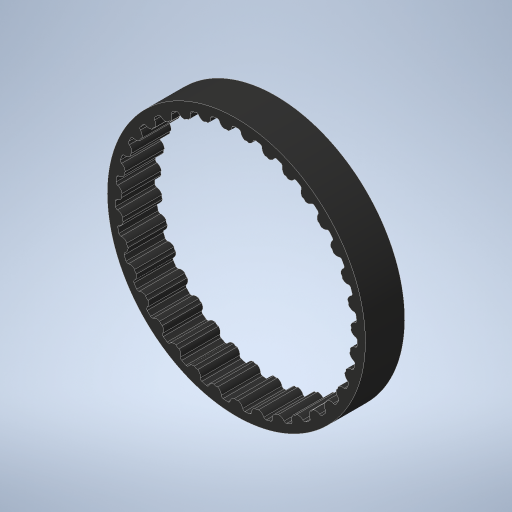
# Autodesk Inventor part: belt tooth
Saved by Autodesk Inventor 2023.3 (Build 273359000, 359)
## iProperties
Created: 2024-02-03
Part Number: belt tooth
Material: Rubber, Silicone
Document SubType Name: Modeling
Designer: mavericks
Density: 1.25 g/cm^3
Appearance: Rubber - Black
Author: mavericks
Autodesk Inventor part; units mm, degrees
ref_plane "YZ Plane" through (0, 0, 0) normal (1, 0, 0) x (0, 1, 0)
ref_plane "XZ Plane" through (0, 0, 0) normal (0, 1, 0) x (-1, 0, 0)
ref_plane "XY Plane" through (0, 0, 0) normal (0, 0, 1) x (1, 0, 0)
sketch "Sketch1" plane through (0, 0, 0) normal (0, 0, 1) x (1, 0, 0)
  line L0 (3.873, 1.9) -> (5, 1.9) construction
  arc A0 (3.3889, 2.275) -> (3.873, 1.9) centre (3.873, 2.4) ccw
  arc A1 (3.3889, 2.275) -> (2.3532, 3.341) centre (1.9365, 1.9) ccw
  arc A2 (1.5198, 3.341) -> (2.3532, 3.341) centre (1.9365, 4.0627) ccw
  arc A3 (1.5198, 3.341) -> (0.4841, 2.275) centre (1.9365, 1.9) ccw
  arc A4 (0, 1.9) -> (0.4841, 2.275) centre (0, 2.4) ccw
  line L1 (0, 0) -> (6.35, 0) construction
  line L2 (0, 1.9) -> (0, 0)
  line L3 (3.873, 1.9) -> (3.873, 0)
  line L4 (3.873, 0) -> (0, 0)
  dimension "d1" = 1.127
  dimension "d2" = 0.5
  dimension "d3" = 1.5
  dimension "d4" = 0.8333
  dimension "d5" = 1.5
  dimension "d6" = 0.5
  dimension "d7" = 1.9
  dimension "d8" = 2.4
  dimension "d9" = 1.9365
  dimension "d10" = 1.9365
  dimension "d11" = 1.6626
  dimension "d12" = 0.5
  dimension "d13" = 1.9
  dimension "d14" = 0
  dimension "d15" = 6.35
  dimension "d16" = 0.4841
  dimension "d17" = 1.0357
  dimension "d18" = 0.375
  dimension "d19" = 1.066
  dimension "Height_of_Tooth" = 3.341
  constraints: 10 end point, 10 point on circle, 5 centre point, 2 perpendicular, 1 coincident, 1 horizontal, 1 point on line
  measures "d1" distance of L0.start L0.end
  measures "d2" radius of A0
  measures "d3" radius of A1
  measures "d4" radius of A2
  measures "d5" radius of A3
  measures "d6" radius of A4
  measures "d7" distance between parallel lines of L1 L0
  measures "d8" distance from line of L1 A4.centre
  measures "d9" horizontal distance of A2.centre A4.centre
  measures "d10" horizontal distance of A0.centre A2.centre
  measures "d11" vertical distance of A2.centre A0.centre
  measures "d12" vertical distance of A1.centre A0.centre
  measures "d13" distance from line of L1 A1.centre
  measures "d14" horizontal distance of L1.start A4.centre
  measures "d15" distance of L1.start L1.end
  measures "d16" horizontal distance of L0.start A0.start
  measures "d17" horizontal distance of A3.end A3.start
  measures "d18" vertical distance of L2.start A3.end
  measures "d19" vertical distance of A3.end A3.start
  measures "Height_of_Tooth" distance from line of L1 A3.start
extrude "Extrusion1" add sketch "Sketch1" along normal mid plane 9
ref_plane "Work Plane1" through (0, 29.5226, 4.5) normal (0, -1, 0) x (1, 0, 0)
sketch "Sketch2" plane through (0, 29.5226, 4.5) normal (0, -1, 0) x (1, 0, 0)
  line L0 (1.5198, -9) -> (1.5198, 0) construction
  line L1 (2.3532, 0) -> (2.3532, 0) construction
  line L2 (2.3532, 0) -> (2.3532, -9) construction
  line L3 (1.5198, -9) -> (2.3532, -9) construction
  line L4 (3.873, -9) -> (0, -9) construction
  line L5 (1.9365, -9) -> (1.9365, 0)
  line L6 (2.3532, 0) -> (2.3532, 0) construction
  point P0 (0, -4.5)
  constraints: 2 end point, 1 midpoint, 1 point on line
pattern_circular "Circular Pattern1" count 35 over 360 about axis through (1.9365, 29.5226, -4.5) along (0, 0, 1) of "Extrusion1"
sketch "Sketch3" plane through (0, 0, 4.5) normal (0, 0, 1) x (1, 0, 0)
  arc A0 (3.3889, 2.275) -> (2.3532, 3.341) centre (1.9365, 1.9) ccw construction
  arc A1 (3.3889, 2.275) -> (3.873, 1.9) centre (3.873, 2.4) ccw construction
  line L0 (3.873, 1.9) -> (3.873, 0) construction
  line L1 (3.873, 0) -> (0, 0) construction
  line L2 (0, 0) -> (0, 1.9) construction
  arc A2 (0, 1.9) -> (0.4841, 2.275) centre (0, 2.4) ccw construction
  arc A3 (1.5198, 3.341) -> (0.4841, 2.275) centre (1.9365, 1.9) ccw construction
  arc A4 (1.5198, 3.341) -> (2.3532, 3.341) centre (1.9365, 4.0627) ccw construction
  arc A5 (8.2308, 2.9722) -> (7.0214, 3.8361) centre (6.8687, 2.3439) ccw construction
  arc A6 (8.2308, 2.9722) -> (8.7741, 2.6897) centre (8.6848, 3.1816) ccw construction
  line L3 (8.7741, 2.6897) -> (9.1133, 0.8202) construction
  line L4 (9.1133, 0.8202) -> (5.3026, 0.1287) construction
  line L5 (5.3026, 0.1287) -> (4.9633, 1.9981) construction
  arc A7 (4.9633, 1.9981) -> (5.3727, 2.4535) centre (4.874, 2.4901) ccw construction
  arc A8 (6.2014, 3.6873) -> (5.3727, 2.4535) centre (6.8687, 2.3439) ccw construction
  arc A9 (6.2014, 3.6873) -> (7.0214, 3.8361) centre (6.4825, 4.4718) ccw construction
  arc A10 (12.8704, 4.5228) -> (11.5262, 5.1568) centre (11.6424, 3.6614) ccw construction
  arc A11 (12.8704, 4.5228) -> (13.4554, 4.3418) centre (13.2797, 4.8099) ccw construction
  line L6 (13.4554, 4.3418) -> (14.123, 2.5629) construction
  line L7 (14.123, 2.5629) -> (10.497, 1.2021) construction
  line L8 (10.497, 1.2021) -> (9.8294, 2.9809) construction
  arc A12 (9.8294, 2.9809) -> (10.1509, 3.5021) centre (9.6537, 3.449) ccw construction
  arc A13 (10.746, 4.864) -> (10.1509, 3.5021) centre (11.6424, 3.6614) ccw construction
  arc A14 (10.746, 4.864) -> (11.5262, 5.1568) centre (10.8825, 5.6861) ccw construction
  arc A15 (17.1585, 6.8768) -> (15.7227, 7.2607) centre (16.1041, 5.81) ccw construction
  arc A16 (17.1585, 6.8768) -> (17.7665, 6.8032) centre (17.51, 7.2325) ccw construction
  line L9 (17.7665, 6.8032) -> (18.741, 5.1722) construction
  line L10 (18.741, 5.1722) -> (15.4162, 3.1857) construction
  line L11 (15.4162, 3.1857) -> (14.4417, 4.8168) construction
  arc A17 (14.4417, 4.8168) -> (14.665, 5.387) centre (14.1853, 5.246) ccw construction
  arc A18 (15.0073, 6.8333) -> (14.665, 5.387) centre (16.1041, 5.81) ccw construction
  arc A19 (15.0073, 6.8333) -> (15.7227, 7.2607) centre (14.9949, 7.6665) ccw construction
  arc A20 (20.9575, 9.9588) -> (19.4762, 10.0801) centre (20.1105, 8.7208) ccw construction
  arc A21 (20.9575, 9.9588) -> (21.5688, 9.9949) centre (21.2398, 10.3714) ccw construction
  line L12 (21.5688, 9.9949) -> (22.8189, 8.5641) construction
  line L13 (22.8189, 8.5641) -> (19.9022, 6.0159) construction
  line L14 (19.9022, 6.0159) -> (18.6522, 7.4467) construction
  arc A22 (18.6522, 7.4467) -> (18.77, 8.0476) centre (18.3232, 7.8233) ccw construction
  arc A23 (18.8486, 9.5318) -> (18.77, 8.0476) centre (20.1105, 8.7208) ccw construction
  arc A24 (18.8486, 9.5318) -> (19.4762, 10.0801) centre (18.6876, 10.3494) ccw construction
  arc A25 (24.1451, 13.6695) -> (22.6659, 13.5244) centre (23.5327, 12.3002) ccw construction
  arc A26 (24.1451, 13.6695) -> (24.7401, 13.8142) centre (24.3492, 14.1259) ccw construction
  line L15 (24.7401, 13.8142) -> (26.2256, 12.6296) construction
  line L16 (26.2256, 12.6296) -> (23.8108, 9.6016) construction
  line L17 (23.8108, 9.6016) -> (22.3253, 10.7862) construction
  arc A27 (22.3253, 10.7862) -> (22.334, 11.3985) centre (21.9344, 11.0979) ccw construction
  arc A28 (22.1463, 12.8729) -> (22.334, 11.3985) centre (23.5327, 12.3002) ccw construction
  arc A29 (22.1463, 12.8729) -> (22.6659, 13.5244) centre (21.8419, 13.6486) ccw construction
  arc A30 (26.6188, 17.8898) -> (25.1894, 17.4829) centre (26.2608, 16.4331) ccw construction
  arc A31 (26.6188, 17.8898) -> (27.1785, 18.1384) centre (26.7382, 18.3753) ccw construction
  line L18 (27.1785, 18.1384) -> (28.8516, 17.238) construction
  line L19 (28.8516, 17.238) -> (27.0163, 13.8275) construction
  line L20 (27.0163, 13.8275) -> (25.3432, 14.7278) construction
  arc A32 (25.3432, 14.7278) -> (25.2424, 15.3319) centre (24.9029, 14.9648) ccw construction
  arc A33 (24.7945, 16.749) -> (25.2424, 15.3319) centre (26.2608, 16.4331) ccw construction
  arc A34 (24.7945, 16.749) -> (25.1894, 17.4829) centre (24.3564, 17.4579) ccw construction
  arc A35 (28.2993, 22.4839) -> (26.9655, 21.8283) centre (28.2071, 20.9867) ccw construction
  arc A36 (28.2993, 22.4839) -> (28.8056, 22.8285) centre (28.33, 22.983) ccw construction
  line L21 (28.8056, 22.8285) -> (30.6126, 22.2413) construction
  line L22 (30.6126, 22.2413) -> (29.4157, 18.5579) construction
  line L23 (29.4157, 18.5579) -> (27.6087, 19.145) construction
  arc A37 (27.6087, 19.145) -> (27.4017, 19.7213) centre (27.1332, 19.2995) ccw construction
  arc A38 (26.7079, 21.0358) -> (27.4017, 19.7213) centre (28.2071, 20.9867) ccw construction
  arc A39 (26.7079, 21.0358) -> (26.9655, 21.8283) centre (26.1503, 21.655) ccw construction
  arc A40 (29.1324, 27.3043) -> (27.9371, 26.421) centre (29.3091, 25.8147) ccw construction
  arc A41 (29.1324, 27.3043) -> (29.569, 27.7337) centre (29.0736, 27.8008) ccw construction
  line L24 (29.569, 27.7337) -> (31.4518, 27.4786) construction
  line L25 (31.4518, 27.4786) -> (30.932, 23.6407) construction
  line L26 (30.932, 23.6407) -> (29.0492, 23.8958) construction
  arc A42 (29.0492, 23.8958) -> (28.7425, 24.4258) centre (28.5537, 23.9629) ccw construction
  arc A43 (27.8252, 25.5953) -> (28.7425, 24.4258) centre (29.3091, 25.8147) ccw construction
  arc A44 (27.8252, 25.5953) -> (27.9371, 26.421) centre (27.166, 26.105) ccw construction
  arc A45 (29.0915, 32.196) -> (28.0731, 31.1135) centre (29.5313, 30.7619) ccw construction
  arc A46 (29.0915, 32.196) -> (29.4444, 32.6964) centre (28.9449, 32.674) ccw construction
  line L27 (29.4444, 32.6964) -> (31.3425, 32.7817) construction
  line L28 (31.3425, 32.7817) -> (31.5162, 28.9126) construction
  line L29 (31.5162, 28.9126) -> (29.6182, 28.8273) construction
  arc A47 (29.6182, 28.8273) -> (29.2218, 29.2942) centre (29.1187, 28.8049) ccw construction
  arc A48 (28.1105, 30.281) -> (29.2218, 29.2942) centre (29.5313, 30.7619) ccw construction
  arc A49 (28.1105, 30.281) -> (28.0731, 31.1135) centre (27.3708, 30.6649) ccw construction
  arc A50 (28.1778, 37.0017) -> (27.369, 35.7548) centre (28.8665, 35.6692) ccw construction
  arc A51 (28.1778, 37.0017) -> (28.4356, 37.5571) centre (27.9482, 37.4459) ccw construction
  line L30 (28.4356, 37.5571) -> (30.288, 37.9799) construction
  line L31 (30.288, 37.9799) -> (31.1498, 34.2041) construction
  line L32 (31.1498, 34.2041) -> (29.2974, 33.7813) construction
  arc A52 (29.2974, 33.7813) -> (28.8241, 34.1698) centre (28.81, 33.67) ccw construction
  arc A53 (27.5544, 34.9423) -> (28.8241, 34.1698) centre (28.8665, 35.6692) ccw construction
  arc A54 (27.5544, 34.9423) -> (27.369, 35.7548) centre (26.7581, 35.188) ccw construction
  arc A55 (26.4206, 41.5671) -> (25.8475, 40.1958) centre (27.3362, 40.379) ccw construction
  arc A56 (26.4206, 41.5671) -> (26.5751, 42.1596) centre (26.1154, 41.9631) ccw construction
  line L33 (26.5751, 42.1596) -> (28.3223, 42.9064) construction
  line L34 (28.3223, 42.9064) -> (29.8444, 39.3451) construction
  line L35 (29.8444, 39.3451) -> (28.0973, 38.5983) construction
  arc A57 (28.0973, 38.5983) -> (27.5622, 38.8961) centre (27.6376, 38.4018) ccw construction
  arc A58 (26.175, 39.4295) -> (27.5622, 38.8961) centre (27.3362, 40.379) ccw construction
  arc A59 (26.175, 39.4295) -> (25.8475, 40.1958) centre (25.3476, 39.529) ccw construction
  arc A60 (23.8765, 45.7453) -> (23.5574, 44.2937) centre (24.9896, 44.7398) ccw construction
  arc A61 (23.8765, 45.7453) -> (23.9228, 46.3559) centre (23.5055, 46.0805) ccw construction
  line L36 (23.9228, 46.3559) -> (25.5085, 47.4027) construction
  line L37 (25.5085, 47.4027) -> (27.6421, 44.1704) construction
  line L38 (27.6421, 44.1704) -> (26.0564, 43.1237) construction
  arc A62 (26.0564, 43.1237) -> (25.4767, 43.3211) centre (25.6391, 42.8482) ccw construction
  arc A63 (24.0165, 43.5982) -> (25.4767, 43.3211) centre (24.9896, 44.7398) ccw construction
  arc A64 (24.0165, 43.5982) -> (23.5574, 44.2937) centre (23.1847, 43.5484) ccw construction
  arc A65 (20.6272, 49.4022) -> (20.5725, 47.9169) centre (21.902, 48.6115) ccw construction
  arc A66 (20.6272, 49.4022) -> (20.5637, 50.0112) centre (20.2023, 49.6657) ccw construction
  line L39 (20.5637, 50.0112) -> (21.937, 51.3242) construction
  line L40 (21.937, 51.3242) -> (24.6135, 48.5249) construction
  line L41 (24.6135, 48.5249) -> (23.2402, 47.2119) construction
  arc A67 (23.2402, 47.2119) -> (22.6346, 47.3026) centre (22.8788, 46.8663) ccw construction
  arc A68 (21.1484, 47.3146) -> (22.6346, 47.3026) centre (21.902, 48.6115) ccw construction
  arc A69 (21.1484, 47.3146) -> (20.5725, 47.9169) centre (20.3388, 47.117) ccw construction
  arc A70 (16.7772, 52.4201) -> (16.9886, 50.9489) centre (18.1726, 51.8698) ccw construction
  arc A71 (16.7772, 52.4201) -> (16.606, 53.008) centre (16.3121, 52.6035) ccw construction
  line L42 (16.606, 53.008) -> (17.7228, 54.5451) construction
  line L43 (17.7228, 54.5451) -> (20.8561, 52.2686) construction
  line L44 (20.8561, 52.2686) -> (19.7393, 50.7315) construction
  arc A72 (19.7393, 50.7315) -> (19.1272, 50.7127) centre (19.4454, 50.327) ccw construction
  arc A73 (17.6628, 50.4591) -> (19.1272, 50.7127) centre (18.1726, 51.8698) ccw construction
  arc A74 (17.6628, 50.4591) -> (16.9886, 50.9489) centre (16.9015, 50.1201) ccw construction
  arc A75 (12.4502, 54.702) -> (12.9209, 53.2922) centre (13.9215, 54.4097) ccw construction
  arc A76 (12.4502, 54.702) -> (12.1768, 55.2499) centre (11.9598, 54.7994) ccw construction
  line L45 (12.1768, 55.2499) -> (13.0011, 56.9618) construction
  line L46 (13.0011, 56.9618) -> (16.4906, 55.2813) construction
  line L47 (16.4906, 55.2813) -> (15.6662, 53.5695) construction
  arc A77 (15.6662, 53.5695) -> (15.0673, 53.4417) centre (15.4493, 53.119) ccw construction
  arc A78 (13.6717, 52.9307) -> (15.0673, 53.4417) centre (13.9215, 54.4097) ccw construction
  arc A79 (13.6717, 52.9307) -> (12.9209, 53.2922) centre (12.9831, 52.4612) ccw construction
  arc A80 (7.7853, 56.1747) -> (8.5001, 54.8716) centre (9.2851, 56.1498) ccw construction
  arc A81 (7.7853, 56.1747) -> (7.4184, 56.6649) centre (7.2854, 56.183) ccw construction
  line L48 (7.4184, 56.6649) -> (7.9239, 58.4965) construction
  line L49 (7.9239, 58.4965) -> (11.6573, 57.4661) construction
  line L50 (11.6573, 57.4661) -> (11.1518, 55.6346) construction
  arc A82 (11.1518, 55.6346) -> (10.5854, 55.4019) centre (11.0188, 55.1526) ccw construction
  arc A83 (9.3034, 54.6499) -> (10.5854, 55.4019) centre (9.2851, 56.1498) ccw construction
  arc A84 (9.3034, 54.6499) -> (8.5001, 54.8716) centre (8.7098, 54.065) ccw construction
  arc A85 (2.9324, 56.7907) -> (3.8684, 55.6362) centre (4.4126, 57.034) ccw construction
  arc A86 (2.9324, 56.7907) -> (2.4839, 57.2076) centre (2.439, 56.7096) ccw construction
  line L51 (2.4839, 57.2076) -> (2.6542, 59.0999) construction
  line L52 (2.6542, 59.0999) -> (6.5116, 58.7528) construction
  line L53 (6.5116, 58.7528) -> (6.3413, 56.8604) construction
  arc A87 (6.3413, 56.8604) -> (5.8255, 56.5303) centre (6.2964, 56.3624) ccw construction
  arc A88 (4.6984, 55.5615) -> (5.8255, 56.5303) centre (4.4126, 57.034) ccw construction
  arc A89 (4.6984, 55.5615) -> (3.8684, 55.6362) centre (4.2187, 54.8801) ccw construction
  arc A90 (-1.9525, 56.5303) -> (-0.8254, 55.5615) centre (-0.5396, 57.034) ccw construction
  arc A91 (-1.9525, 56.5303) -> (-2.4683, 56.8604) centre (-2.4235, 56.3624) ccw construction
  line L54 (-2.4683, 56.8604) -> (-2.6386, 58.7528) construction
  line L55 (-2.6386, 58.7528) -> (1.2188, 59.0999) construction
  line L56 (1.2188, 59.0999) -> (1.3891, 57.2076) construction
  arc A92 (1.3891, 57.2076) -> (0.9406, 56.7907) centre (1.4339, 56.7096) ccw construction
  arc A93 (0.0046, 55.6362) -> (0.9406, 56.7907) centre (-0.5396, 57.034) ccw construction
  arc A94 (0.0046, 55.6362) -> (-0.8254, 55.5615) centre (-0.3457, 54.8801) ccw construction
  arc A95 (-6.7124, 55.4019) -> (-5.4304, 54.6499) centre (-5.4121, 56.1498) ccw construction
  arc A96 (-6.7124, 55.4019) -> (-7.2788, 55.6346) centre (-7.1458, 55.1526) ccw construction
  line L57 (-7.2788, 55.6346) -> (-7.7843, 57.4661) construction
  line L58 (-7.7843, 57.4661) -> (-4.0509, 58.4965) construction
  line L59 (-4.0509, 58.4965) -> (-3.5454, 56.6649) construction
  arc A97 (-3.5454, 56.6649) -> (-3.9123, 56.1747) centre (-3.4124, 56.183) ccw construction
  arc A98 (-4.6271, 54.8716) -> (-3.9123, 56.1747) centre (-5.4121, 56.1498) ccw construction
  arc A99 (-4.6271, 54.8716) -> (-5.4304, 54.6499) centre (-4.8368, 54.065) ccw construction
  arc A100 (-11.1943, 53.4417) -> (-9.7987, 52.9307) centre (-10.0485, 54.4097) ccw construction
  arc A101 (-11.1943, 53.4417) -> (-11.7932, 53.5695) centre (-11.5763, 53.119) ccw construction
  line L60 (-11.7932, 53.5695) -> (-12.6176, 55.2813) construction
  line L61 (-12.6176, 55.2813) -> (-9.1282, 56.9618) construction
  line L62 (-9.1282, 56.9618) -> (-8.3038, 55.2499) construction
  arc A102 (-8.3038, 55.2499) -> (-8.5773, 54.702) centre (-8.0868, 54.7994) ccw construction
  arc A103 (-9.0479, 53.2922) -> (-8.5773, 54.702) centre (-10.0485, 54.4097) ccw construction
  arc A104 (-9.0479, 53.2922) -> (-9.7987, 52.9307) centre (-9.1102, 52.4612) ccw construction
  arc A105 (-15.2542, 50.7127) -> (-13.7898, 50.4591) centre (-14.2997, 51.8698) ccw construction
  arc A106 (-15.2542, 50.7127) -> (-15.8663, 50.7315) centre (-15.5724, 50.327) ccw construction
  line L63 (-15.8663, 50.7315) -> (-16.9831, 52.2686) construction
  line L64 (-16.9831, 52.2686) -> (-13.8498, 54.5451) construction
  line L65 (-13.8498, 54.5451) -> (-12.733, 53.008) construction
  arc A107 (-12.733, 53.008) -> (-12.9043, 52.4201) centre (-12.4391, 52.6035) ccw construction
  arc A108 (-13.1156, 50.9489) -> (-12.9043, 52.4201) centre (-14.2997, 51.8698) ccw construction
  arc A109 (-13.1156, 50.9489) -> (-13.7898, 50.4591) centre (-13.0285, 50.1201) ccw construction
  arc A110 (-18.7616, 47.3026) -> (-17.2754, 47.3146) centre (-18.029, 48.6115) ccw construction
  arc A111 (-18.7616, 47.3026) -> (-19.3672, 47.2119) centre (-19.0058, 46.8663) ccw construction
  line L66 (-19.3672, 47.2119) -> (-20.7405, 48.5249) construction
  line L67 (-20.7405, 48.5249) -> (-18.0641, 51.3242) construction
  line L68 (-18.0641, 51.3242) -> (-16.6907, 50.0112) construction
  arc A112 (-16.6907, 50.0112) -> (-16.7543, 49.4022) centre (-16.3293, 49.6657) ccw construction
  arc A113 (-16.6995, 47.9169) -> (-16.7543, 49.4022) centre (-18.029, 48.6115) ccw construction
  arc A114 (-16.6995, 47.9169) -> (-17.2754, 47.3146) centre (-16.4658, 47.117) ccw construction
  arc A115 (-21.6037, 43.3211) -> (-20.1435, 43.5982) centre (-21.1166, 44.7398) ccw construction
  arc A116 (-21.6037, 43.3211) -> (-22.1834, 43.1237) centre (-21.7661, 42.8482) ccw construction
  line L69 (-22.1834, 43.1237) -> (-23.7691, 44.1704) construction
  line L70 (-23.7691, 44.1704) -> (-21.6355, 47.4027) construction
  line L71 (-21.6355, 47.4027) -> (-20.0498, 46.3559) construction
  arc A117 (-20.0498, 46.3559) -> (-20.0035, 45.7453) centre (-19.6325, 46.0805) ccw construction
  arc A118 (-19.6845, 44.2937) -> (-20.0035, 45.7453) centre (-21.1166, 44.7398) ccw construction
  arc A119 (-19.6845, 44.2937) -> (-20.1435, 43.5982) centre (-19.3117, 43.5484) ccw construction
  arc A120 (-23.6893, 38.8961) -> (-22.302, 39.4295) centre (-23.4633, 40.379) ccw construction
  arc A121 (-23.6893, 38.8961) -> (-24.2243, 38.5983) centre (-23.7646, 38.4018) ccw construction
  line L72 (-24.2243, 38.5983) -> (-25.9714, 39.3451) construction
  line L73 (-25.9714, 39.3451) -> (-24.4493, 42.9064) construction
  line L74 (-24.4493, 42.9064) -> (-22.7022, 42.1596) construction
  arc A122 (-22.7022, 42.1596) -> (-22.5476, 41.5671) centre (-22.2424, 41.9631) ccw construction
  arc A123 (-21.9745, 40.1958) -> (-22.5476, 41.5671) centre (-23.4633, 40.379) ccw construction
  arc A124 (-21.9745, 40.1958) -> (-22.302, 39.4295) centre (-21.4746, 39.529) ccw construction
  arc A125 (-24.9511, 34.1698) -> (-23.6814, 34.9423) centre (-24.9936, 35.6692) ccw construction
  arc A126 (-24.9511, 34.1698) -> (-25.4245, 33.7813) centre (-24.937, 33.67) ccw construction
  line L75 (-25.4245, 33.7813) -> (-27.2768, 34.2041) construction
  line L76 (-27.2768, 34.2041) -> (-26.415, 37.9799) construction
  line L77 (-26.415, 37.9799) -> (-24.5626, 37.5571) construction
  arc A127 (-24.5626, 37.5571) -> (-24.3048, 37.0017) centre (-24.0752, 37.4459) ccw construction
  arc A128 (-23.496, 35.7548) -> (-24.3048, 37.0017) centre (-24.9936, 35.6692) ccw construction
  arc A129 (-23.496, 35.7548) -> (-23.6814, 34.9423) centre (-22.8851, 35.188) ccw construction
  arc A130 (-25.3488, 29.2942) -> (-24.2375, 30.281) centre (-25.6583, 30.7619) ccw construction
  arc A131 (-25.3488, 29.2942) -> (-25.7452, 28.8273) centre (-25.2457, 28.8049) ccw construction
  line L78 (-25.7452, 28.8273) -> (-27.6433, 28.9126) construction
  line L79 (-27.6433, 28.9126) -> (-27.4695, 32.7817) construction
  line L80 (-27.4695, 32.7817) -> (-25.5714, 32.6964) construction
  arc A132 (-25.5714, 32.6964) -> (-25.2185, 32.196) centre (-25.0719, 32.674) ccw construction
  arc A133 (-24.2001, 31.1135) -> (-25.2185, 32.196) centre (-25.6583, 30.7619) ccw construction
  arc A134 (-24.2001, 31.1135) -> (-24.2375, 30.281) centre (-23.4978, 30.6649) ccw construction
  arc A135 (-24.8696, 24.4258) -> (-23.9523, 25.5953) centre (-25.4361, 25.8147) ccw construction
  arc A136 (-24.8696, 24.4258) -> (-25.1762, 23.8958) centre (-24.6807, 23.9629) ccw construction
  line L81 (-25.1762, 23.8958) -> (-27.059, 23.6407) construction
  line L82 (-27.059, 23.6407) -> (-27.5789, 27.4786) construction
  line L83 (-27.5789, 27.4786) -> (-25.6961, 27.7337) construction
  arc A137 (-25.6961, 27.7337) -> (-25.2595, 27.3043) centre (-25.2006, 27.8008) ccw construction
  arc A138 (-24.0641, 26.421) -> (-25.2595, 27.3043) centre (-25.4361, 25.8147) ccw construction
  arc A139 (-24.0641, 26.421) -> (-23.9523, 25.5953) centre (-23.293, 26.105) ccw construction
  arc A140 (-23.5287, 19.7213) -> (-22.835, 21.0358) centre (-24.3342, 20.9867) ccw construction
  arc A141 (-23.5287, 19.7213) -> (-23.7358, 19.145) centre (-23.2602, 19.2995) ccw construction
  line L84 (-23.7358, 19.145) -> (-25.5428, 18.5579) construction
  line L85 (-25.5428, 18.5579) -> (-26.7396, 22.2413) construction
  line L86 (-26.7396, 22.2413) -> (-24.9326, 22.8285) construction
  arc A142 (-24.9326, 22.8285) -> (-24.4263, 22.4839) centre (-24.457, 22.983) ccw construction
  arc A143 (-23.0925, 21.8283) -> (-24.4263, 22.4839) centre (-24.3342, 20.9867) ccw construction
  arc A144 (-23.0925, 21.8283) -> (-22.835, 21.0358) centre (-22.2774, 21.655) ccw construction
  arc A145 (-21.3694, 15.3319) -> (-20.9215, 16.749) centre (-22.3878, 16.4331) ccw construction
  arc A146 (-21.3694, 15.3319) -> (-21.4702, 14.7278) centre (-21.0299, 14.9648) ccw construction
  line L87 (-21.4702, 14.7278) -> (-23.1433, 13.8275) construction
  line L88 (-23.1433, 13.8275) -> (-24.9786, 17.238) construction
  line L89 (-24.9786, 17.238) -> (-23.3055, 18.1384) construction
  arc A147 (-23.3055, 18.1384) -> (-22.7459, 17.8898) centre (-22.8652, 18.3753) ccw construction
  arc A148 (-21.3164, 17.4829) -> (-22.7459, 17.8898) centre (-22.3878, 16.4331) ccw construction
  arc A149 (-21.3164, 17.4829) -> (-20.9215, 16.749) centre (-20.4834, 17.4579) ccw construction
  arc A150 (-18.461, 11.3985) -> (-18.2733, 12.8729) centre (-19.6597, 12.3002) ccw construction
  arc A151 (-18.461, 11.3985) -> (-18.4523, 10.7862) centre (-18.0614, 11.0979) ccw construction
  line L90 (-18.4523, 10.7862) -> (-19.9378, 9.6016) construction
  line L91 (-19.9378, 9.6016) -> (-22.3526, 12.6296) construction
  line L92 (-22.3526, 12.6296) -> (-20.8671, 13.8142) construction
  arc A152 (-20.8671, 13.8142) -> (-20.2721, 13.6695) centre (-20.4762, 14.1259) ccw construction
  arc A153 (-18.7929, 13.5244) -> (-20.2721, 13.6695) centre (-19.6597, 12.3002) ccw construction
  arc A154 (-18.7929, 13.5244) -> (-18.2733, 12.8729) centre (-17.9689, 13.6486) ccw construction
  arc A155 (-14.897, 8.0476) -> (-14.9756, 9.5318) centre (-16.2375, 8.7208) ccw construction
  arc A156 (-14.897, 8.0476) -> (-14.7792, 7.4467) centre (-14.4502, 7.8233) ccw construction
  line L93 (-14.7792, 7.4467) -> (-16.0293, 6.0159) construction
  line L94 (-16.0293, 6.0159) -> (-18.9459, 8.5641) construction
  line L95 (-18.9459, 8.5641) -> (-17.6958, 9.9949) construction
  arc A157 (-17.6958, 9.9949) -> (-17.0845, 9.9588) centre (-17.3668, 10.3714) ccw construction
  arc A158 (-15.6032, 10.0801) -> (-17.0845, 9.9588) centre (-16.2375, 8.7208) ccw construction
  arc A159 (-15.6032, 10.0801) -> (-14.9756, 9.5318) centre (-14.8146, 10.3494) ccw construction
  arc A160 (-10.792, 5.387) -> (-11.1344, 6.8333) centre (-12.2311, 5.81) ccw construction
  arc A161 (-10.792, 5.387) -> (-10.5687, 4.8168) centre (-10.3123, 5.246) ccw construction
  line L96 (-10.5687, 4.8168) -> (-11.5433, 3.1857) construction
  line L97 (-11.5433, 3.1857) -> (-14.868, 5.1722) construction
  line L98 (-14.868, 5.1722) -> (-13.8935, 6.8032) construction
  arc A162 (-13.8935, 6.8032) -> (-13.2856, 6.8768) centre (-13.637, 7.2325) ccw construction
  arc A163 (-11.8497, 7.2607) -> (-13.2856, 6.8768) centre (-12.2311, 5.81) ccw construction
  arc A164 (-11.8497, 7.2607) -> (-11.1344, 6.8333) centre (-11.1219, 7.6665) ccw construction
  arc A165 (-6.2779, 3.5021) -> (-6.873, 4.864) centre (-7.7694, 3.6614) ccw construction
  arc A166 (-6.2779, 3.5021) -> (-5.9564, 2.9809) centre (-5.7807, 3.449) ccw construction
  line L99 (-5.9564, 2.9809) -> (-6.624, 1.2021) construction
  line L100 (-6.624, 1.2021) -> (-10.25, 2.5629) construction
  line L101 (-10.25, 2.5629) -> (-9.5824, 4.3418) construction
  arc A167 (-9.5824, 4.3418) -> (-8.9974, 4.5228) centre (-9.4067, 4.8099) ccw construction
  arc A168 (-7.6532, 5.1568) -> (-8.9974, 4.5228) centre (-7.7694, 3.6614) ccw construction
  arc A169 (-7.6532, 5.1568) -> (-6.873, 4.864) centre (-7.0095, 5.6861) ccw construction
  arc A170 (-1.4997, 2.4535) -> (-2.3285, 3.6873) centre (-2.9957, 2.3439) ccw construction
  arc A171 (-1.4997, 2.4535) -> (-1.0903, 1.9981) centre (-1.0011, 2.4901) ccw construction
  line L102 (-1.0903, 1.9981) -> (-1.4296, 0.1287) construction
  line L103 (-1.4296, 0.1287) -> (-5.2403, 0.8202) construction
  line L104 (-5.2403, 0.8202) -> (-4.9011, 2.6897) construction
  arc A172 (-4.9011, 2.6897) -> (-4.3578, 2.9722) centre (-4.8118, 3.1816) ccw construction
  arc A173 (-3.1484, 3.8361) -> (-4.3578, 2.9722) centre (-2.9957, 2.3439) ccw construction
  arc A174 (-3.1484, 3.8361) -> (-2.3285, 3.6873) centre (-2.6096, 4.4718) ccw construction
  arc A175 (3.3889, 2.275) -> (2.3532, 3.341) centre (1.9365, 1.9) ccw construction
  arc A176 (3.3889, 2.275) -> (3.873, 1.9) centre (3.873, 2.4) ccw construction
  line L105 (3.873, 1.9) -> (3.873, 0) construction
  line L106 (3.873, 0) -> (0, 0) construction
  line L107 (0, 0) -> (0, 1.9) construction
  arc A177 (0, 1.9) -> (0.4841, 2.275) centre (0, 2.4) ccw construction
  arc A178 (1.5198, 3.341) -> (0.4841, 2.275) centre (1.9365, 1.9) ccw construction
  arc A179 (1.5198, 3.341) -> (2.3532, 3.341) centre (1.9365, 4.0627) ccw construction
  circle A180 centre (1.9365, 29.5226) radius 29.5226
  circle A181 centre (1.9365, 29.5226) radius 27.6904
  circle A182 centre (1.9365, 29.5226) radius 32.6976
  arc A183 (8.2308, 2.9722) -> (7.0214, 3.8361) centre (6.8687, 2.3439) ccw projected
  arc A184 (8.2308, 2.9722) -> (8.7741, 2.6897) centre (8.6848, 3.1816) ccw projected
  line L108 (8.7741, 2.6897) -> (9.1133, 0.8202) projected
  line L109 (9.1133, 0.8202) -> (5.3026, 0.1287) projected
  line L110 (5.3026, 0.1287) -> (4.9633, 1.9981) projected
  arc A185 (4.9633, 1.9981) -> (5.3727, 2.4535) centre (4.874, 2.4901) ccw projected
  arc A186 (6.2014, 3.6873) -> (5.3727, 2.4535) centre (6.8687, 2.3439) ccw projected
  arc A187 (6.2014, 3.6873) -> (7.0214, 3.8361) centre (6.4825, 4.4718) ccw projected
  arc A188 (12.8704, 4.5228) -> (11.5262, 5.1568) centre (11.6424, 3.6614) ccw projected
  arc A189 (12.8704, 4.5228) -> (13.4554, 4.3418) centre (13.2797, 4.8099) ccw projected
  line L111 (13.4554, 4.3418) -> (14.123, 2.5629) projected
  line L112 (14.123, 2.5629) -> (10.497, 1.2021) projected
  line L113 (10.497, 1.2021) -> (9.8294, 2.9809) projected
  arc A190 (9.8294, 2.9809) -> (10.1509, 3.5021) centre (9.6537, 3.449) ccw projected
  arc A191 (10.746, 4.864) -> (10.1509, 3.5021) centre (11.6424, 3.6614) ccw projected
  arc A192 (10.746, 4.864) -> (11.5262, 5.1568) centre (10.8825, 5.6861) ccw projected
  arc A193 (17.1585, 6.8768) -> (15.7227, 7.2607) centre (16.1041, 5.81) ccw projected
  arc A194 (17.1585, 6.8768) -> (17.7665, 6.8032) centre (17.51, 7.2325) ccw projected
  line L114 (17.7665, 6.8032) -> (18.741, 5.1722) projected
  line L115 (18.741, 5.1722) -> (15.4162, 3.1857) projected
  line L116 (15.4162, 3.1857) -> (14.4417, 4.8168) projected
  arc A195 (14.4417, 4.8168) -> (14.665, 5.387) centre (14.1853, 5.246) ccw projected
  arc A196 (15.0073, 6.8333) -> (14.665, 5.387) centre (16.1041, 5.81) ccw projected
  arc A197 (15.0073, 6.8333) -> (15.7227, 7.2607) centre (14.9949, 7.6665) ccw projected
  arc A198 (20.9575, 9.9588) -> (19.4762, 10.0801) centre (20.1105, 8.7208) ccw projected
  arc A199 (20.9575, 9.9588) -> (21.5688, 9.9949) centre (21.2398, 10.3714) ccw projected
  line L117 (21.5688, 9.9949) -> (22.8189, 8.5641) projected
  line L118 (22.8189, 8.5641) -> (19.9022, 6.0159) projected
  line L119 (19.9022, 6.0159) -> (18.6522, 7.4467) projected
  arc A200 (18.6522, 7.4467) -> (18.77, 8.0476) centre (18.3232, 7.8233) ccw projected
  arc A201 (18.8486, 9.5318) -> (18.77, 8.0476) centre (20.1105, 8.7208) ccw projected
  arc A202 (18.8486, 9.5318) -> (19.4762, 10.0801) centre (18.6876, 10.3494) ccw projected
  arc A203 (24.1451, 13.6695) -> (22.6659, 13.5244) centre (23.5327, 12.3002) ccw projected
  arc A204 (24.1451, 13.6695) -> (24.7401, 13.8142) centre (24.3492, 14.1259) ccw projected
  line L120 (24.7401, 13.8142) -> (26.2256, 12.6296) projected
  line L121 (26.2256, 12.6296) -> (23.8108, 9.6016) projected
  line L122 (23.8108, 9.6016) -> (22.3253, 10.7862) projected
  arc A205 (22.3253, 10.7862) -> (22.334, 11.3985) centre (21.9344, 11.0979) ccw projected
  arc A206 (22.1463, 12.8729) -> (22.334, 11.3985) centre (23.5327, 12.3002) ccw projected
  arc A207 (22.1463, 12.8729) -> (22.6659, 13.5244) centre (21.8419, 13.6486) ccw projected
  arc A208 (26.6188, 17.8898) -> (25.1894, 17.4829) centre (26.2608, 16.4331) ccw projected
  arc A209 (26.6188, 17.8898) -> (27.1785, 18.1384) centre (26.7382, 18.3753) ccw projected
  line L123 (27.1785, 18.1384) -> (28.8516, 17.238) projected
  line L124 (28.8516, 17.238) -> (27.0163, 13.8275) projected
  line L125 (27.0163, 13.8275) -> (25.3432, 14.7278) projected
  arc A210 (25.3432, 14.7278) -> (25.2424, 15.3319) centre (24.9029, 14.9648) ccw projected
  arc A211 (24.7945, 16.749) -> (25.2424, 15.3319) centre (26.2608, 16.4331) ccw projected
  arc A212 (24.7945, 16.749) -> (25.1894, 17.4829) centre (24.3564, 17.4579) ccw projected
  arc A213 (28.2993, 22.4839) -> (26.9655, 21.8283) centre (28.2071, 20.9867) ccw projected
  arc A214 (28.2993, 22.4839) -> (28.8056, 22.8285) centre (28.33, 22.983) ccw projected
  line L126 (28.8056, 22.8285) -> (30.6126, 22.2413) projected
  line L127 (30.6126, 22.2413) -> (29.4157, 18.5579) projected
  line L128 (29.4157, 18.5579) -> (27.6087, 19.145) projected
  arc A215 (27.6087, 19.145) -> (27.4017, 19.7213) centre (27.1332, 19.2995) ccw projected
  arc A216 (26.7079, 21.0358) -> (27.4017, 19.7213) centre (28.2071, 20.9867) ccw projected
  arc A217 (26.7079, 21.0358) -> (26.9655, 21.8283) centre (26.1503, 21.655) ccw projected
  arc A218 (29.1324, 27.3043) -> (27.9371, 26.421) centre (29.3091, 25.8147) ccw projected
  arc A219 (29.1324, 27.3043) -> (29.569, 27.7337) centre (29.0736, 27.8008) ccw projected
  line L129 (29.569, 27.7337) -> (31.4518, 27.4786) projected
  line L130 (31.4518, 27.4786) -> (30.932, 23.6407) projected
  line L131 (30.932, 23.6407) -> (29.0492, 23.8958) projected
  arc A220 (29.0492, 23.8958) -> (28.7425, 24.4258) centre (28.5537, 23.9629) ccw projected
  arc A221 (27.8252, 25.5953) -> (28.7425, 24.4258) centre (29.3091, 25.8147) ccw projected
  arc A222 (27.8252, 25.5953) -> (27.9371, 26.421) centre (27.166, 26.105) ccw projected
  arc A223 (29.0915, 32.196) -> (28.0731, 31.1135) centre (29.5313, 30.7619) ccw projected
  arc A224 (29.0915, 32.196) -> (29.4444, 32.6964) centre (28.9449, 32.674) ccw projected
  line L132 (29.4444, 32.6964) -> (31.3425, 32.7817) projected
  line L133 (31.3425, 32.7817) -> (31.5162, 28.9126) projected
  line L134 (31.5162, 28.9126) -> (29.6182, 28.8273) projected
  arc A225 (29.6182, 28.8273) -> (29.2218, 29.2942) centre (29.1187, 28.8049) ccw projected
  arc A226 (28.1105, 30.281) -> (29.2218, 29.2942) centre (29.5313, 30.7619) ccw projected
  arc A227 (28.1105, 30.281) -> (28.0731, 31.1135) centre (27.3708, 30.6649) ccw projected
  arc A228 (28.1778, 37.0017) -> (27.369, 35.7548) centre (28.8665, 35.6692) ccw projected
  arc A229 (28.1778, 37.0017) -> (28.4356, 37.5571) centre (27.9482, 37.4459) ccw projected
  line L135 (28.4356, 37.5571) -> (30.288, 37.9799) projected
  line L136 (30.288, 37.9799) -> (31.1498, 34.2041) projected
  line L137 (31.1498, 34.2041) -> (29.2974, 33.7813) projected
  arc A230 (29.2974, 33.7813) -> (28.8241, 34.1698) centre (28.81, 33.67) ccw projected
  arc A231 (27.5544, 34.9423) -> (28.8241, 34.1698) centre (28.8665, 35.6692) ccw projected
  arc A232 (27.5544, 34.9423) -> (27.369, 35.7548) centre (26.7581, 35.188) ccw projected
  arc A233 (26.4206, 41.5671) -> (25.8475, 40.1958) centre (27.3362, 40.379) ccw projected
  arc A234 (26.4206, 41.5671) -> (26.5751, 42.1596) centre (26.1154, 41.9631) ccw projected
  line L138 (26.5751, 42.1596) -> (28.3223, 42.9064) projected
  line L139 (28.3223, 42.9064) -> (29.8444, 39.3451) projected
  line L140 (29.8444, 39.3451) -> (28.0973, 38.5983) projected
  arc A235 (28.0973, 38.5983) -> (27.5622, 38.8961) centre (27.6376, 38.4018) ccw projected
  arc A236 (26.175, 39.4295) -> (27.5622, 38.8961) centre (27.3362, 40.379) ccw projected
  arc A237 (26.175, 39.4295) -> (25.8475, 40.1958) centre (25.3476, 39.529) ccw projected
  arc A238 (23.8765, 45.7453) -> (23.5574, 44.2937) centre (24.9896, 44.7398) ccw projected
  arc A239 (23.8765, 45.7453) -> (23.9228, 46.3559) centre (23.5055, 46.0805) ccw projected
  line L141 (23.9228, 46.3559) -> (25.5085, 47.4027) projected
  line L142 (25.5085, 47.4027) -> (27.6421, 44.1704) projected
  line L143 (27.6421, 44.1704) -> (26.0564, 43.1237) projected
  arc A240 (26.0564, 43.1237) -> (25.4767, 43.3211) centre (25.6391, 42.8482) ccw projected
  arc A241 (24.0165, 43.5982) -> (25.4767, 43.3211) centre (24.9896, 44.7398) ccw projected
  arc A242 (24.0165, 43.5982) -> (23.5574, 44.2937) centre (23.1847, 43.5484) ccw projected
  arc A243 (20.6272, 49.4022) -> (20.5725, 47.9169) centre (21.902, 48.6115) ccw projected
  arc A244 (20.6272, 49.4022) -> (20.5637, 50.0112) centre (20.2023, 49.6657) ccw projected
  line L144 (20.5637, 50.0112) -> (21.937, 51.3242) projected
  line L145 (21.937, 51.3242) -> (24.6135, 48.5249) projected
  line L146 (24.6135, 48.5249) -> (23.2402, 47.2119) projected
  arc A245 (23.2402, 47.2119) -> (22.6346, 47.3026) centre (22.8788, 46.8663) ccw projected
  arc A246 (21.1484, 47.3146) -> (22.6346, 47.3026) centre (21.902, 48.6115) ccw projected
  arc A247 (21.1484, 47.3146) -> (20.5725, 47.9169) centre (20.3388, 47.117) ccw projected
  arc A248 (16.7772, 52.4201) -> (16.9886, 50.9489) centre (18.1726, 51.8698) ccw projected
  arc A249 (16.7772, 52.4201) -> (16.606, 53.008) centre (16.3121, 52.6035) ccw projected
  line L147 (16.606, 53.008) -> (17.7228, 54.5451) projected
  line L148 (17.7228, 54.5451) -> (20.8561, 52.2686) projected
  line L149 (20.8561, 52.2686) -> (19.7393, 50.7315) projected
  arc A250 (19.7393, 50.7315) -> (19.1272, 50.7127) centre (19.4454, 50.327) ccw projected
  arc A251 (17.6628, 50.4591) -> (19.1272, 50.7127) centre (18.1726, 51.8698) ccw projected
  arc A252 (17.6628, 50.4591) -> (16.9886, 50.9489) centre (16.9015, 50.1201) ccw projected
  arc A253 (12.4502, 54.702) -> (12.9209, 53.2922) centre (13.9215, 54.4097) ccw projected
  arc A254 (12.4502, 54.702) -> (12.1768, 55.2499) centre (11.9598, 54.7994) ccw projected
  line L150 (12.1768, 55.2499) -> (13.0011, 56.9618) projected
  line L151 (13.0011, 56.9618) -> (16.4906, 55.2813) projected
  line L152 (16.4906, 55.2813) -> (15.6662, 53.5695) projected
  arc A255 (15.6662, 53.5695) -> (15.0673, 53.4417) centre (15.4493, 53.119) ccw projected
  arc A256 (13.6717, 52.9307) -> (15.0673, 53.4417) centre (13.9215, 54.4097) ccw projected
  arc A257 (13.6717, 52.9307) -> (12.9209, 53.2922) centre (12.9831, 52.4612) ccw projected
  arc A258 (7.7853, 56.1747) -> (8.5001, 54.8716) centre (9.2851, 56.1498) ccw projected
  arc A259 (7.7853, 56.1747) -> (7.4184, 56.6649) centre (7.2854, 56.183) ccw projected
  line L153 (7.4184, 56.6649) -> (7.9239, 58.4965) projected
  line L154 (7.9239, 58.4965) -> (11.6573, 57.4661) projected
  line L155 (11.6573, 57.4661) -> (11.1518, 55.6346) projected
  arc A260 (11.1518, 55.6346) -> (10.5854, 55.4019) centre (11.0188, 55.1526) ccw projected
  arc A261 (9.3034, 54.6499) -> (10.5854, 55.4019) centre (9.2851, 56.1498) ccw projected
  arc A262 (9.3034, 54.6499) -> (8.5001, 54.8716) centre (8.7098, 54.065) ccw projected
  arc A263 (2.9324, 56.7907) -> (3.8684, 55.6362) centre (4.4126, 57.034) ccw projected
  arc A264 (2.9324, 56.7907) -> (2.4839, 57.2076) centre (2.439, 56.7096) ccw projected
  line L156 (2.4839, 57.2076) -> (2.6542, 59.0999) projected
  line L157 (2.6542, 59.0999) -> (6.5116, 58.7528) projected
  line L158 (6.5116, 58.7528) -> (6.3413, 56.8604) projected
  arc A265 (6.3413, 56.8604) -> (5.8255, 56.5303) centre (6.2964, 56.3624) ccw projected
  arc A266 (4.6984, 55.5615) -> (5.8255, 56.5303) centre (4.4126, 57.034) ccw projected
  arc A267 (4.6984, 55.5615) -> (3.8684, 55.6362) centre (4.2187, 54.8801) ccw projected
  arc A268 (-1.9525, 56.5303) -> (-0.8254, 55.5615) centre (-0.5396, 57.034) ccw projected
  arc A269 (-1.9525, 56.5303) -> (-2.4683, 56.8604) centre (-2.4235, 56.3624) ccw projected
  line L159 (-2.4683, 56.8604) -> (-2.6386, 58.7528) projected
  line L160 (-2.6386, 58.7528) -> (1.2188, 59.0999) projected
  line L161 (1.2188, 59.0999) -> (1.3891, 57.2076) projected
  arc A270 (1.3891, 57.2076) -> (0.9406, 56.7907) centre (1.4339, 56.7096) ccw projected
  arc A271 (0.0046, 55.6362) -> (0.9406, 56.7907) centre (-0.5396, 57.034) ccw projected
  arc A272 (0.0046, 55.6362) -> (-0.8254, 55.5615) centre (-0.3457, 54.8801) ccw projected
  arc A273 (-6.7124, 55.4019) -> (-5.4304, 54.6499) centre (-5.4121, 56.1498) ccw projected
  arc A274 (-6.7124, 55.4019) -> (-7.2788, 55.6346) centre (-7.1458, 55.1526) ccw projected
  line L162 (-7.2788, 55.6346) -> (-7.7843, 57.4661) projected
  line L163 (-7.7843, 57.4661) -> (-4.0509, 58.4965) projected
  line L164 (-4.0509, 58.4965) -> (-3.5454, 56.6649) projected
  arc A275 (-3.5454, 56.6649) -> (-3.9123, 56.1747) centre (-3.4124, 56.183) ccw projected
  arc A276 (-4.6271, 54.8716) -> (-3.9123, 56.1747) centre (-5.4121, 56.1498) ccw projected
  arc A277 (-4.6271, 54.8716) -> (-5.4304, 54.6499) centre (-4.8368, 54.065) ccw projected
  arc A278 (-11.1943, 53.4417) -> (-9.7987, 52.9307) centre (-10.0485, 54.4097) ccw projected
  arc A279 (-11.1943, 53.4417) -> (-11.7932, 53.5695) centre (-11.5763, 53.119) ccw projected
  line L165 (-11.7932, 53.5695) -> (-12.6176, 55.2813) projected
  line L166 (-12.6176, 55.2813) -> (-9.1282, 56.9618) projected
  line L167 (-9.1282, 56.9618) -> (-8.3038, 55.2499) projected
  arc A280 (-8.3038, 55.2499) -> (-8.5773, 54.702) centre (-8.0868, 54.7994) ccw projected
  arc A281 (-9.0479, 53.2922) -> (-8.5773, 54.702) centre (-10.0485, 54.4097) ccw projected
  arc A282 (-9.0479, 53.2922) -> (-9.7987, 52.9307) centre (-9.1102, 52.4612) ccw projected
  arc A283 (-15.2542, 50.7127) -> (-13.7898, 50.4591) centre (-14.2997, 51.8698) ccw projected
  arc A284 (-15.2542, 50.7127) -> (-15.8663, 50.7315) centre (-15.5724, 50.327) ccw projected
  line L168 (-15.8663, 50.7315) -> (-16.9831, 52.2686) projected
  line L169 (-16.9831, 52.2686) -> (-13.8498, 54.5451) projected
  line L170 (-13.8498, 54.5451) -> (-12.733, 53.008) projected
  arc A285 (-12.733, 53.008) -> (-12.9043, 52.4201) centre (-12.4391, 52.6035) ccw projected
  arc A286 (-13.1156, 50.9489) -> (-12.9043, 52.4201) centre (-14.2997, 51.8698) ccw projected
  arc A287 (-13.1156, 50.9489) -> (-13.7898, 50.4591) centre (-13.0285, 50.1201) ccw projected
  arc A288 (-18.7616, 47.3026) -> (-17.2754, 47.3146) centre (-18.029, 48.6115) ccw projected
  arc A289 (-18.7616, 47.3026) -> (-19.3672, 47.2119) centre (-19.0058, 46.8663) ccw projected
  line L171 (-19.3672, 47.2119) -> (-20.7405, 48.5249) projected
  line L172 (-20.7405, 48.5249) -> (-18.0641, 51.3242) projected
  line L173 (-18.0641, 51.3242) -> (-16.6907, 50.0112) projected
  arc A290 (-16.6907, 50.0112) -> (-16.7543, 49.4022) centre (-16.3293, 49.6657) ccw projected
  arc A291 (-16.6995, 47.9169) -> (-16.7543, 49.4022) centre (-18.029, 48.6115) ccw projected
  arc A292 (-16.6995, 47.9169) -> (-17.2754, 47.3146) centre (-16.4658, 47.117) ccw projected
  arc A293 (-21.6037, 43.3211) -> (-20.1435, 43.5982) centre (-21.1166, 44.7398) ccw projected
  arc A294 (-21.6037, 43.3211) -> (-22.1834, 43.1237) centre (-21.7661, 42.8482) ccw projected
  line L174 (-22.1834, 43.1237) -> (-23.7691, 44.1704) projected
  line L175 (-23.7691, 44.1704) -> (-21.6355, 47.4027) projected
  line L176 (-21.6355, 47.4027) -> (-20.0498, 46.3559) projected
  arc A295 (-20.0498, 46.3559) -> (-20.0035, 45.7453) centre (-19.6325, 46.0805) ccw projected
  arc A296 (-19.6845, 44.2937) -> (-20.0035, 45.7453) centre (-21.1166, 44.7398) ccw projected
  arc A297 (-19.6845, 44.2937) -> (-20.1435, 43.5982) centre (-19.3117, 43.5484) ccw projected
  arc A298 (-23.6893, 38.8961) -> (-22.302, 39.4295) centre (-23.4633, 40.379) ccw projected
  arc A299 (-23.6893, 38.8961) -> (-24.2243, 38.5983) centre (-23.7646, 38.4018) ccw projected
  line L177 (-24.2243, 38.5983) -> (-25.9714, 39.3451) projected
  line L178 (-25.9714, 39.3451) -> (-24.4493, 42.9064) projected
  line L179 (-24.4493, 42.9064) -> (-22.7022, 42.1596) projected
  arc A300 (-22.7022, 42.1596) -> (-22.5476, 41.5671) centre (-22.2424, 41.9631) ccw projected
  arc A301 (-21.9745, 40.1958) -> (-22.5476, 41.5671) centre (-23.4633, 40.379) ccw projected
  arc A302 (-21.9745, 40.1958) -> (-22.302, 39.4295) centre (-21.4746, 39.529) ccw projected
  arc A303 (-24.9511, 34.1698) -> (-23.6814, 34.9423) centre (-24.9936, 35.6692) ccw projected
  arc A304 (-24.9511, 34.1698) -> (-25.4245, 33.7813) centre (-24.937, 33.67) ccw projected
  line L180 (-25.4245, 33.7813) -> (-27.2768, 34.2041) projected
  line L181 (-27.2768, 34.2041) -> (-26.415, 37.9799) projected
  line L182 (-26.415, 37.9799) -> (-24.5626, 37.5571) projected
  arc A305 (-24.5626, 37.5571) -> (-24.3048, 37.0017) centre (-24.0752, 37.4459) ccw projected
  arc A306 (-23.496, 35.7548) -> (-24.3048, 37.0017) centre (-24.9936, 35.6692) ccw projected
  arc A307 (-23.496, 35.7548) -> (-23.6814, 34.9423) centre (-22.8851, 35.188) ccw projected
  arc A308 (-25.3488, 29.2942) -> (-24.2375, 30.281) centre (-25.6583, 30.7619) ccw projected
  arc A309 (-25.3488, 29.2942) -> (-25.7452, 28.8273) centre (-25.2457, 28.8049) ccw projected
  line L183 (-25.7452, 28.8273) -> (-27.6433, 28.9126) projected
  line L184 (-27.6433, 28.9126) -> (-27.4695, 32.7817) projected
  line L185 (-27.4695, 32.7817) -> (-25.5714, 32.6964) projected
  arc A310 (-25.5714, 32.6964) -> (-25.2185, 32.196) centre (-25.0719, 32.674) ccw projected
  arc A311 (-24.2001, 31.1135) -> (-25.2185, 32.196) centre (-25.6583, 30.7619) ccw projected
  arc A312 (-24.2001, 31.1135) -> (-24.2375, 30.281) centre (-23.4978, 30.6649) ccw projected
  arc A313 (-24.8696, 24.4258) -> (-23.9523, 25.5953) centre (-25.4361, 25.8147) ccw projected
  arc A314 (-24.8696, 24.4258) -> (-25.1762, 23.8958) centre (-24.6807, 23.9629) ccw projected
  line L186 (-25.1762, 23.8958) -> (-27.059, 23.6407) projected
  line L187 (-27.059, 23.6407) -> (-27.5789, 27.4786) projected
  line L188 (-27.5789, 27.4786) -> (-25.6961, 27.7337) projected
  arc A315 (-25.6961, 27.7337) -> (-25.2595, 27.3043) centre (-25.2006, 27.8008) ccw projected
  arc A316 (-24.0641, 26.421) -> (-25.2595, 27.3043) centre (-25.4361, 25.8147) ccw projected
  arc A317 (-24.0641, 26.421) -> (-23.9523, 25.5953) centre (-23.293, 26.105) ccw projected
  arc A318 (-23.5287, 19.7213) -> (-22.835, 21.0358) centre (-24.3342, 20.9867) ccw projected
  arc A319 (-23.5287, 19.7213) -> (-23.7358, 19.145) centre (-23.2602, 19.2995) ccw projected
  line L189 (-23.7358, 19.145) -> (-25.5428, 18.5579) projected
  line L190 (-25.5428, 18.5579) -> (-26.7396, 22.2413) projected
  line L191 (-26.7396, 22.2413) -> (-24.9326, 22.8285) projected
  arc A320 (-24.9326, 22.8285) -> (-24.4263, 22.4839) centre (-24.457, 22.983) ccw projected
  arc A321 (-23.0925, 21.8283) -> (-24.4263, 22.4839) centre (-24.3342, 20.9867) ccw projected
  arc A322 (-23.0925, 21.8283) -> (-22.835, 21.0358) centre (-22.2774, 21.655) ccw projected
  arc A323 (-21.3694, 15.3319) -> (-20.9215, 16.749) centre (-22.3878, 16.4331) ccw projected
  arc A324 (-21.3694, 15.3319) -> (-21.4702, 14.7278) centre (-21.0299, 14.9648) ccw projected
  line L192 (-21.4702, 14.7278) -> (-23.1433, 13.8275) projected
  line L193 (-23.1433, 13.8275) -> (-24.9786, 17.238) projected
  line L194 (-24.9786, 17.238) -> (-23.3055, 18.1384) projected
  arc A325 (-23.3055, 18.1384) -> (-22.7459, 17.8898) centre (-22.8652, 18.3753) ccw projected
  arc A326 (-21.3164, 17.4829) -> (-22.7459, 17.8898) centre (-22.3878, 16.4331) ccw projected
  arc A327 (-21.3164, 17.4829) -> (-20.9215, 16.749) centre (-20.4834, 17.4579) ccw projected
  arc A328 (-18.461, 11.3985) -> (-18.2733, 12.8729) centre (-19.6597, 12.3002) ccw projected
  arc A329 (-18.461, 11.3985) -> (-18.4523, 10.7862) centre (-18.0614, 11.0979) ccw projected
  line L195 (-18.4523, 10.7862) -> (-19.9378, 9.6016) projected
  line L196 (-19.9378, 9.6016) -> (-22.3526, 12.6296) projected
  line L197 (-22.3526, 12.6296) -> (-20.8671, 13.8142) projected
  arc A330 (-20.8671, 13.8142) -> (-20.2721, 13.6695) centre (-20.4762, 14.1259) ccw projected
  arc A331 (-18.7929, 13.5244) -> (-20.2721, 13.6695) centre (-19.6597, 12.3002) ccw projected
  arc A332 (-18.7929, 13.5244) -> (-18.2733, 12.8729) centre (-17.9689, 13.6486) ccw projected
  arc A333 (-14.897, 8.0476) -> (-14.9756, 9.5318) centre (-16.2375, 8.7208) ccw projected
  arc A334 (-14.897, 8.0476) -> (-14.7792, 7.4467) centre (-14.4502, 7.8233) ccw projected
  line L198 (-14.7792, 7.4467) -> (-16.0293, 6.0159) projected
  line L199 (-16.0293, 6.0159) -> (-18.9459, 8.5641) projected
  line L200 (-18.9459, 8.5641) -> (-17.6958, 9.9949) projected
  arc A335 (-17.6958, 9.9949) -> (-17.0845, 9.9588) centre (-17.3668, 10.3714) ccw projected
  arc A336 (-15.6032, 10.0801) -> (-17.0845, 9.9588) centre (-16.2375, 8.7208) ccw projected
  arc A337 (-15.6032, 10.0801) -> (-14.9756, 9.5318) centre (-14.8146, 10.3494) ccw projected
  arc A338 (-10.792, 5.387) -> (-11.1344, 6.8333) centre (-12.2311, 5.81) ccw projected
  arc A339 (-10.792, 5.387) -> (-10.5687, 4.8168) centre (-10.3123, 5.246) ccw projected
  line L201 (-10.5687, 4.8168) -> (-11.5433, 3.1857) projected
  line L202 (-11.5433, 3.1857) -> (-14.868, 5.1722) projected
  line L203 (-14.868, 5.1722) -> (-13.8935, 6.8032) projected
  arc A340 (-13.8935, 6.8032) -> (-13.2856, 6.8768) centre (-13.637, 7.2325) ccw projected
  arc A341 (-11.8497, 7.2607) -> (-13.2856, 6.8768) centre (-12.2311, 5.81) ccw projected
  arc A342 (-11.8497, 7.2607) -> (-11.1344, 6.8333) centre (-11.1219, 7.6665) ccw projected
  arc A343 (-6.2779, 3.5021) -> (-6.873, 4.864) centre (-7.7694, 3.6614) ccw projected
  arc A344 (-6.2779, 3.5021) -> (-5.9564, 2.9809) centre (-5.7807, 3.449) ccw projected
  line L204 (-5.9564, 2.9809) -> (-6.624, 1.2021) projected
  line L205 (-6.624, 1.2021) -> (-10.25, 2.5629) projected
  line L206 (-10.25, 2.5629) -> (-9.5824, 4.3418) projected
  arc A345 (-9.5824, 4.3418) -> (-8.9974, 4.5228) centre (-9.4067, 4.8099) ccw projected
  arc A346 (-7.6532, 5.1568) -> (-8.9974, 4.5228) centre (-7.7694, 3.6614) ccw projected
  arc A347 (-7.6532, 5.1568) -> (-6.873, 4.864) centre (-7.0095, 5.6861) ccw projected
  arc A348 (-1.4997, 2.4535) -> (-2.3285, 3.6873) centre (-2.9957, 2.3439) ccw projected
  arc A349 (-1.4997, 2.4535) -> (-1.0903, 1.9981) centre (-1.0011, 2.4901) ccw projected
  line L207 (-1.0903, 1.9981) -> (-1.4296, 0.1287) projected
  line L208 (-1.4296, 0.1287) -> (-5.2403, 0.8202) projected
  line L209 (-5.2403, 0.8202) -> (-4.9011, 2.6897) projected
  arc A350 (-4.9011, 2.6897) -> (-4.3578, 2.9722) centre (-4.8118, 3.1816) ccw projected
  arc A351 (-3.1484, 3.8361) -> (-4.3578, 2.9722) centre (-2.9957, 2.3439) ccw projected
  arc A352 (-3.1484, 3.8361) -> (-2.3285, 3.6873) centre (-2.6096, 4.4718) ccw projected
  dimension "d26" = 59.0452
  dimension "d27" = 3.175
  constraints: 3 coincident, 2 centre point, 3 other
  measures "d26" diameter of A180
  measures "d27" radial gap between concentric circles of A180 A182
extrude "Extrusion2" add sketch "Sketch3" against normal up to surface (9 mm away) contours A180 L134 A181 L132 | A180 L129 A181 L134 | L132 A181 L137 A180 | A180 L131 A181 L129 | L137 A181 L135 A180 | A180 L126 A181 L131 | L135 A181 L140 A180 | A180 L128 A181 L126 | L140 A181 L138 A180 | L128 A180 L123 A181 | A181 L143 A180 L138 | L123 A180 L125 A181 | A181 L141 A180 L143 | L125 A180 L120 A181 | A181 L146 A180 L141 | L120 A180 L122 A181 | A181 L144 A180 L146 | L122 A180 L117 A181 | A181 L149 A180 L144 | L117 A180 L119 A181 | A181 L147 A180 L149 | L119 A180 L114 A181 | A181 L152 A180 L147 | L114 A180 L116 A181 | A181 L150 A180 L152 | L116 A180 L111 A181 | A181 L155 A180 L150 | L111 A180 L113 A181 | A181 L153 A180 L155 | L113 A180 L108 A181 | A181 L158 A180 L153 | L108 A180 L110 A181 | A181 L156 A180 L158 | L110 A180 L207 A181 | A181 L161 A180 L156 | L207 A180 L209 A181 | A181 L159 A180 L161 | L209 A180 L204 A181 | A181 L164 A180 L159 | L204 A180 L206 A181 | A181 L162 A180 L164 | L206 A180 L201 A181 | A181 L167 A180 L162 | L201 A180 L203 A181 | A181 L165 A180 L167 | L203 A180 L198 A181 | A181 L170 A180 L165 | L198 A180 L200 A181 | A181 L168 A180 L170 | L200 A180 L195 A181 | A181 L173 A180 L168 | L195 A180 L197 A181 | A181 L171 A180 L173 | L197 A180 L192 A181 | A181 L176 A180 L171 | L192 A180 L194 A181 | A181 L174 A180 L176 | L194 A180 L189 A181 | A181 L179 A180 L174 | L189 A180 L191 A181 | A181 L177 A180 L179 | L191 A180 L186 A181 | A181 L182 A180 L177 | L186 A180 L188 A181 | A181 L180 A180 L182 | L188 A180 L183 A181 | A181 L185 A180 L180 | L183 A180 L185 A181
extrude "Extrusion3" cut sketch "Sketch3" against normal up to surface (9 mm away) contours A180 L133 L134 | A180 L132 L133 | L129 L130 A180 | A180 L136 L137 | L130 L131 A180 | A180 L135 L136 | L126 L127 A180 | A180 L139 L140 | L127 L128 A180 | A180 L138 L139 | L123 L124 A180 | A180 L142 L143 | L124 L125 A180 | A180 L141 L142 | L120 L121 A180 | A180 L145 L146 | A180 L121 L122 | L144 L145 A180 | L117 L118 A180 | A180 L148 L149 | A180 L118 L119 | L147 L148 A180 | L114 L115 A180 | A180 L151 L152 | A180 L115 L116 | L150 L151 A180 | L111 L112 A180 | A180 L154 L155 | A180 L112 L113 | L153 L154 A180 | L108 L109 A180 | A180 L157 L158 | A180 L109 L110 | L156 L157 A180 | L207 L208 A180 | A180 L160 L161 | A180 L208 L209 | L159 L160 A180 | L204 L205 A180 | A180 L163 L164 | A180 L205 L206 | L162 L163 A180 | L201 L202 A180 | A180 L166 L167 | A180 L202 L203 | L165 L166 A180 | L198 L199 A180 | A180 L169 L170 | A180 L199 L200 | L168 L169 A180 | L195 L196 A180 | A180 L172 L173 | A180 L196 L197 | L171 L172 A180 | L192 L193 A180 | A180 L175 L176 | A180 L193 L194 | L174 L175 A180 | L189 L190 A180 | A180 L178 L179 | A180 L190 L191 | L177 L178 A180 | L186 L187 A180 | A180 L181 L182 | A180 L187 L188 | L180 L181 A180 | L183 L184 A180 | A180 L184 L185 | A182
equation "\"Height_Teeth_half\" = 0.5 * Height_of_Tooth"
body "Solid1"
